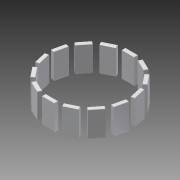
# Autodesk Inventor part: magnets
Saved by Autodesk Inventor 2012 (Build 160160000, 160)
## iProperties
Created: 2014-07-09
Part Number: magnets
Material: Default
Document SubType Name: Modeling
Designer: Anon
Density: 1 g/cm^3
Author: Anon
Autodesk Inventor part; units mm, degrees
ref_plane "YZ Plane" through (0, 0, 0) normal (1, 0, 0) x (0, 1, 0)
ref_plane "XZ Plane" through (0, 0, 0) normal (0, 1, 0) x (-1, 0, 0)
ref_plane "XY Plane" through (0, 0, 0) normal (0, 0, 1) x (1, 0, 0)
sketch "Sketch1" plane through (0, 0, 0) normal (0, 0, 1) x (1, 0, 0)
  line L0 (-2.5, 16.5) -> (2.5, 16.5)
  line L1 (2.5, 16.5) -> (2.5, 15)
  line L2 (2.5, 15) -> (-2.5, 15)
  line L3 (-2.5, 15) -> (-2.5, 16.5)
  point P0 (0, 0)
  dimension "d0" = 5
  dimension "d1" = 2.5
  dimension "d2" = 1.5
  dimension "d3" = 15
  constraints: 8 end point, 2 parallel, 1 horizontal, 1 perpendicular
  measures "d0" distance between parallel lines of L1 L3
  measures "d1" distance from line of point (0, 0) L3
  measures "d2" distance between parallel lines of L2 L0
  measures "d3" distance from line of point (0, 0) L2
extrude "Extrusion1" add sketch "Sketch1" along normal blind 10
fillet "Fillet1" radius 0.2 8 edges at (-2.5, 15.75, 10) (0, 16.5, 10) (0, 15, 10) (2.5, 15.75, 10) (0, 15, 0) (-2.5, 15.75, 0) (0, 16.5, 0) (2.5, 15.75, 0)
pattern_circular "Circular Pattern1" count 14 over 360 about axis through (0, 0, -10) along (0, 0, 1) of "Extrusion1", "Fillet1"
body "Solid1"
